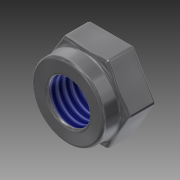
# Autodesk Inventor part: NylstopNut_M3
Saved by Autodesk Inventor 2014 SP1 (Build 180222100, 222)
## iProperties
Created: 2015-03-29
Part Number: NylstopNut_M3
Material: Generic
Document SubType Name: Modeling
Designer: david
Density: 1 g/cm^3
Appearance: Default
Author: david
Autodesk Inventor part; units mm, degrees
ref_plane "YZ Plane" through (0, 0, 0) normal (1, 0, 0) x (0, 1, 0)
ref_plane "XZ Plane" through (0, 0, 0) normal (0, 1, 0) x (-1, 0, 0)
ref_plane "XY Plane" through (0, 0, 0) normal (0, 0, 1) x (1, 0, 0)
sketch "Sketch1" plane through (0, 0, 0) normal (0, 1, 0) x (-1, 0, 0)
  circle A0 centre (0, 0) radius 1.5
  line L0 (3.1754, 0) -> (1.5877, -2.75)
  line L1 (1.5877, -2.75) -> (-1.5877, -2.75)
  line L2 (-1.5877, -2.75) -> (-3.1754, 0)
  line L3 (-3.1754, 0) -> (-1.5877, 2.75)
  line L4 (-1.5877, 2.75) -> (1.5877, 2.75)
  line L5 (1.5877, 2.75) -> (3.1754, 0)
  dimension "d0" = 3
  dimension "d1" = 5.5
  constraints: 12 end point, 2 coincident, 1 centre point, 13 other
  measures "d0" diameter of A0
  measures "d1" distance between parallel lines of L0 L3
extrude "Extrusion1" add sketch "Sketch1" along normal blind 2
sketch "Sketch2" plane through (0, 0, 0) normal (0, -1, 0) x (1, 0, 0)
  circle A0 centre (0, 0) radius 1.5 projected
  circle A1 centre (0, 0) radius 2.6
  dimension "d13" = 5.2
  constraints: 1 centre point, 1 coincident
  measures "d13" diameter of A1
extrude "Extrusion2" add sketch "Sketch2" along normal blind 1.25
fillet "Fillet1" radius 0.2 22 edges at (-2.6, 0, 0) (-2.6, -1.25, 0) (-1.5, -1.25, 0) (3.1754, 1, 0) (1.5877, 1, -2.75) (-1.5877, 1, -2.75) (-1.5877, 1, 2.75) (-3.1754, 1, 0) (1.5877, 1, 2.75) (1.5, 2, 0) (-2.3816, 0, 1.375) (0, 0, 2.75) (2.3816, 0, 1.375) (2.3816, 0, -1.375) (0, 0, -2.75) (-2.3816, 0, -1.375) (-2.3816, 2, -1.375) (-2.3816, 2, 1.375) (0, 2, 2.75) (2.3816, 2, 1.375) (2.3816, 2, -1.375) (0, 2, -2.75)
thread "Thread1" size "M3x0.5" class "6H" standard "ANSI Metric M Profile" full length
body "Solid1"
